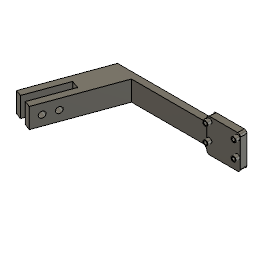
Camera+Arm (Autodesk Fusion 360 design; units mm, degrees)
Autodesk Fusion 360 part; units mm, degrees
sketch "Sketch1" plane through (0, 0, 0) normal (0, 0, 1) x (1, 0, 0)
  circle A0 centre (10.5, -3.138) radius 1.2
  line L0 (-10.5, 12.5) -> (10.5, 12.5)
  arc A1 (-12.5, -10.5) -> (-10.5, -12.5) centre (-10.5, -10.5) ccw
  circle A2 centre (-10.5, -3.138) radius 1.2
  arc A3 (10.5, -12.5) -> (12.5, -10.5) centre (10.5, -10.5) ccw
  circle A4 centre (-10.5, 9.362) radius 1.2
  arc A5 (-10.5, 12.5) -> (-12.5, 10.5) centre (-10.5, 10.5) ccw
  line L1 (-12.5, -10.5) -> (-12.5, 10.5)
  line L2 (12.5, 10.5) -> (12.5, -10.5)
  arc A6 (12.5, 10.5) -> (10.5, 12.5) centre (10.5, 10.5) ccw
  circle A7 centre (10.5, 9.362) radius 1.2
  line L3 (10.5, -12.5) -> (-10.5, -12.5)
  point P0 (-12.5, 12.5)
  point P1 (12.5, 12.5)
  point P2 (-12.5, -12.5)
  dimension "d1" = 25
  dimension "d2" = 25
  dimension "d3" = 2.4
  dimension "d4" = 2
  dimension "d5" = 2
  dimension "d6" = 2
  dimension "d7" = 2
  dimension "d8" = 2
  dimension "d9" = 2
  dimension "d10" = 2
  dimension "d11" = 12.5
  dimension "d12" = 12.5
  dimension "d13" = 21.862
  dimension "d14" = 21.862
  dimension "d15" = 9.362
  dimension "d16" = 9.362
  dimension "d17" = 12.5
  dimension "d18" = 12.5
  constraint horizontal L0
  constraint vertical L2
  constraint horizontal L3
  constraint vertical L1
  constraint equal A2 A4
  constraint equal A0 A2
  constraint equal A0 A7
  constraint coincident P0 L0
  constraint coincident P0 L1
  constraint tangent L0 A5
  constraint tangent A5 L1
  constraint coincident P1 L0
  constraint coincident P1 L2
  constraint tangent L0 A6
  constraint tangent L2 A6
  constraint equal A5 A6
  constraint coincident P2 L3
  constraint coincident P2 L1
  constraint tangent A1 L3
  constraint tangent A1 L1
  constraint tangent A3 L2
  constraint tangent A3 L3
  measures "d1" distance of P0 P1
  measures "d2" distance of P0 P2
  measures "d3" diameter of A4
  measures "d4" distance of A7.centre L2
  measures "d5" distance of A0.centre L2
  measures "d6" distance of A2.centre L1
  measures "d7" distance of A4.centre L1
  measures "d8" radius of A5
  measures "d9" radius of A1
  measures "d10" radius of A3
  measures "d11" distance of origin L1
  measures "d12" distance of origin L0
  measures "d13" distance of A7.centre L3
  measures "d14" distance of A4.centre L3
  measures "d15" distance of A0.centre L3
  measures "d16" distance of A2.centre L3
  measures "d17" distance of origin L1
  measures "d18" distance of origin L0
extrude "Extrude1" add sketch "Sketch1" along normal blind 5
sketch "Sketch2" plane through (0, 0, 5) normal (0, 0, 1) x (1, 0, 0)
  circle A0 centre (-10.5, 9.362) radius 1.2
  circle A1 centre (10.5, -3.138) radius 1.2
  circle A2 centre (-10.5, -3.138) radius 1.2
  circle A3 centre (10.5, 9.362) radius 1.2
  arc A4 (12.5, 10.5) -> (10.5, 12.5) centre (10.5, 10.5) ccw
  line L0 (10.5, 12.5) -> (-10.5, 12.5)
  arc A5 (-10.5, 12.5) -> (-12.5, 10.5) centre (-10.5, 10.5) ccw
  line L1 (-12.5, 10.5) -> (-12.5, -10.5)
  arc A6 (-12.5, -10.5) -> (-10.5, -12.5) centre (-10.5, -10.5) ccw
  line L2 (-10.5, -12.5) -> (10.5, -12.5)
  arc A7 (10.5, -12.5) -> (12.5, -10.5) centre (10.5, -10.5) ccw
  line L3 (12.5, -10.5) -> (12.5, 10.5)
  circle A8 centre (-10.5, 9.362) radius 1.85
  circle A9 centre (10.5, 9.362) radius 1.85
  circle A10 centre (10.5, -3.138) radius 1.85
  circle A11 centre (-10.5, -3.138) radius 1.85
  dimension "d21" = 3.7
  dimension "d22" = 3.7
  dimension "d23" = 3.7
  dimension "d24" = 3.7
  constraint concentric A0 A8
  constraint concentric A3 A9
  constraint concentric A1 A10
  constraint concentric A2 A11
  measures "d21" diameter of A8
  measures "d22" diameter of A9
  measures "d23" diameter of A10
  measures "d24" diameter of A11
extrude "Extrude2" add sketch "Sketch2" along normal blind 3 contours A8 | A9 | A10 | A11
sketch "Sketch3" plane through (-12.5, 0, 0) normal (-1, 0, 0) x (0, 0, 1)
  line L0 (0, 10.5) -> (0, -10.5)
  line L1 (0, -10.5) -> (5, -10.5)
  line L2 (5, -10.5) -> (5, 10.5)
  line L3 (5, 10.5) -> (0, 10.5)
  line L4 (0, 7.5) -> (5, 7.5)
  line L5 (5, 7.5) -> (5, -7.5)
  line L6 (5, -7.5) -> (0, -7.5)
  line L7 (0, -7.5) -> (0, 7.5)
  dimension "d29" = 3
  dimension "d30" = 3
  constraint horizontal L4
  constraint vertical L5
  constraint horizontal L6
  constraint vertical L7
  constraint coincident L2 L5.end
  constraint coincident L0 L4.start
  measures "d29" distance of L3 L4
  measures "d30" distance of L1 L6
extrude "Extrude3" add sketch "Sketch3" along normal blind 68 contours L0 L2 L4 L5 L6 L7
fillet "Fillet1" radius 3 2 edges at (-12.5, 7.5, 2.5) (-12.5, -7.5, 2.5)
sketch "Sketch5" plane through (0, 7.5, 0) normal (0, 1, 0) x (-1, 0, 0)
  line L0 (15.5, 5) -> (15.5, 0)
  line L1 (15.5, 0) -> (80.5, 0)
  line L2 (80.5, 0) -> (80.5, 5)
  line L3 (80.5, 5) -> (15.5, 5)
  line L4 (80.5, 0) -> (94.2374, 0)
  line L5 (94.2374, 0) -> (80.5, 5)
  line L6 (84.001, 0) -> (85.1985, 3.2899)
  dimension "d38" = 20
  dimension "d39" = 5
  dimension "d40" = 5
  constraint coincident L1.end L2.start
  constraint perpendicular L2 L4
  constraint coincident L2.end L3.start
  constraint coincident L4 L6.start
  constraint coincident L5 L6.end
  constraint perpendicular L5 L6
  measures "d38" angle of L4 L5
  measures "d39" distance of L1.end L2.end
  measures "d40" distance of L2.end L6.end
extrude "Extrude5" add sketch "Sketch5" against normal up to surface (15 mm away) contours L2 L4 L5 L6
sketch "Sketch6" plane through (-11.0237, 0, 30.2873) normal (-0.34202, 0, 0.939693) x (0.939693, 0, 0.34202)
  line L0 (-78.9352, -7.5) -> (-73.9352, -7.5)
  line L1 (-73.9352, -7.5) -> (-73.9352, 7.5)
  line L2 (-73.9352, 7.5) -> (-78.9352, 7.5)
  line L3 (-78.9352, 7.5) -> (-78.9352, -7.5)
  line L4 (-78.9352, 7.5) -> (-73.9352, 7.5)
  line L5 (-73.9352, 7.5) -> (-73.9352, -7.5)
  line L6 (-73.9352, -7.5) -> (-78.9352, -7.5)
  line L7 (-78.9352, -7.5) -> (-78.9352, 7.5)
  constraint horizontal L4
  constraint vertical L5
  constraint horizontal L6
  constraint vertical L7
  constraint coincident L0.end L1.start
  constraint coincident L2.end L3.start
extrude "Extrude6" add sketch "Sketch6" along normal blind 55.398
sketch "Sketch7" plane through (-69.4763, 0, -25.2873) normal (0.939693, 0, 0.34202) x (0.34202, 0, -0.939693)
  line L0 (-32.2311, -7.5) -> (-32.2311, 7.5)
  line L1 (-32.2311, 7.5) -> (-87.6291, 7.5)
  line L2 (-87.6291, 7.5) -> (-87.6291, -7.5)
  line L3 (-87.6291, -7.5) -> (-32.2311, -7.5)
  line L4 (-87.6291, 0) -> (-32.2311, 0) construction
  circle A0 centre (-80.1291, 0) radius 2.25
  circle A1 centre (-70.1291, 0) radius 2.25
  dimension "d45" = 4.5
  dimension "d46" = 4.5
  dimension "d47" = 7.5
  dimension "d48" = 10
  constraint midpoint L2 L4.start
  constraint midpoint L0 L4.end
  constraint coincident L4 A0.centre
  constraint coincident L4 A1.centre
  measures "d45" diameter of A0
  measures "d46" diameter of A1
  measures "d47" distance of L2 A0.centre
  measures "d48" distance of A0.centre A1.centre
extrude "Extrude7" cut sketch "Sketch7" against normal up to surface (5 mm away) contours A0 | A1
sketch "Sketch8" plane through (0, 7.5, 0) normal (0, 1, 0) x (-1, 0, 0)
  line L0 (15.5, 5) -> (15.5, 0)
  line L1 (15.5, 0) -> (84.001, 0)
  line L2 (84.001, 0) -> (104.1457, 55.347)
  line L3 (104.1457, 55.347) -> (99.4472, 57.0571)
  line L4 (99.4472, 57.0571) -> (80.5, 5)
  line L5 (80.5, 5) -> (15.5, 5)
  line L6 (74.0085, 5) -> (93.7151, 59.1434)
  line L7 (93.7151, 59.1434) -> (89.0166, 60.8535)
  line L8 (89.0166, 60.8535) -> (68.6876, 5)
  line L9 (99.4472, 57.0571) -> (93.7151, 59.1434) construction
  dimension "d51" = 6.1
  dimension "d52" = 5
  constraint coincident L5 L6.start
  constraint perpendicular L6 L7
  constraint coincident L5 L8.end
  constraint parallel L4 L6
  constraint perpendicular L7 L8
  constraint coincident L3.end L4.start
  constraint perpendicular L4 L9
  measures "d51" distance of L4 L6
  measures "d52" distance of L6.end L7.end
extrude "Extrude8" add sketch "Sketch8" against normal up to surface (15 mm away) contours L5 L6 L7 L8
sketch "Sketch9" plane through (-59.0457, 0, -21.4909) normal (0.939693, 0, 0.34202) x (0.34202, 0, -0.939693)
  line L0 (-87.6291, -7.5) -> (-28.191, -7.5)
  line L1 (-28.191, -7.5) -> (-28.191, 7.5)
  line L2 (-28.191, 7.5) -> (-87.6291, 7.5)
  line L3 (-87.6291, 7.5) -> (-87.6291, -7.5)
  circle A0 centre (-80.1291, 0) radius 2.25
  circle A1 centre (-70.1291, 0) radius 2.25
extrude "Extrude9" cut sketch "Sketch9" against normal up to surface (5 mm away) contours A0 | A1
sketch "Sketch10" plane through (0, 7.5, 0) normal (0, 1, 0) x (-1, 0, 0)
  line L0 (15.5, 5) -> (15.5, 0)
  line L1 (15.5, 0) -> (84.001, 0)
  line L2 (84.001, 0) -> (104.1457, 55.347)
  line L3 (104.1457, 55.347) -> (99.4472, 57.0571)
  line L4 (99.4472, 57.0571) -> (80.5, 5)
  line L5 (80.5, 5) -> (74.0085, 5)
  line L6 (74.0085, 5) -> (93.7151, 59.1434)
  line L7 (93.7151, 59.1434) -> (89.0166, 60.8535)
  line L8 (89.0166, 60.8535) -> (68.6876, 5)
  line L9 (68.6876, 5) -> (15.5, 5)
  line L10 (89.0505, 28.4923) -> (83.3184, 30.5786)
  dimension "d57" = 30.398
  constraint coincident L4 L10.start
  constraint coincident L6 L10.end
  constraint perpendicular L6 L10
  measures "d57" distance of L3 L10
extrude "Extrude10" add sketch "Sketch10" against normal up to surface (15 mm away) contours L4 L5 L6 L10
equation "d17 = d11"
equation "d18 = d12"
equation "d22 = d21"
equation "d23 = d21"
equation "d24 = d21"
equation "d30 = d29"
equation "d40 = d39"
equation "d43 = 19.898 mm + 7.5 mm + 28 mm"
equation "d46 = d45"
equation "d57 = d43 - 25 mm"
